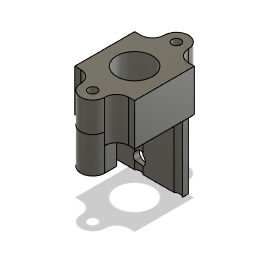
Miniscope_v4_Excitation (Autodesk Fusion 360 design; units mm, degrees)
Autodesk Fusion 360 part; units mm, degrees
sketch "Sketch1" plane through (0, 0, 0) normal (0, 1, 0) x (1, 0, 0)
  line L0 (-1.75, -2.5) -> (1.75, -2.5)
  line L1 (1.75, -2.5) -> (1.75, 2.5)
  line L2 (1.75, 2.5) -> (-1.75, 2.5)
  line L3 (-1.75, 2.5) -> (-1.75, -2.5)
  line L4 (-1.75, -2.5) -> (1.75, 2.5) construction
  line L5 (1.75, -2.5) -> (-1.75, 2.5) construction
  dimension "d1" = 5
  dimension "d2" = 3.5
  constraint perpendicular L0 L1
  constraint parallel L0 L2
  constraint parallel L1 L3
  constraint horizontal L0
  constraint coincident L4 origin
  constraint coincident L5 origin
  measures "d1" distance of L0.end L1.end
  measures "d2" distance of L1.end L2.end
sketch "Sketch2" plane through (0, 0, 0) normal (0, 1, 0) x (1, 0, 0)
  line L0 (-2.5, -2.5) -> (2.5, -2.5)
  line L1 (2.5, -2.5) -> (2.5, 2.5)
  line L2 (2.5, 2.5) -> (-2.5, 2.5)
  line L3 (-2.5, 2.5) -> (-2.5, -2.5)
  line L4 (-2.5, -2.5) -> (2.5, 2.5) construction
  line L5 (2.5, -2.5) -> (-2.5, 2.5) construction
  dimension "d5" = 5
  dimension "d6" = 5
  constraint perpendicular L0 L1
  constraint parallel L0 L2
  constraint parallel L1 L3
  constraint horizontal L0
  constraint coincident L4 origin
  constraint coincident L5 origin
  measures "d5" distance of L1.end L2.end
  measures "d6" distance of L0.end L1.end
extrude "Extrude2" add sketch "Sketch2" along normal blind 3.5
sketch "Sketch3" plane through (0, 3.5, 0) normal (0, 1, 0) x (-1, 0, 0)
  line L0 (2.5, -2.5) -> (2.5, 2.5)
  line L1 (2.5, 2.5) -> (-2.5, 2.5)
  line L2 (-2.5, 2.5) -> (-2.5, -2.5)
  line L3 (-2.5, -2.5) -> (2.5, -2.5)
  circle A0 centre (0, 0) radius 1.5
  dimension "d9" = 3
  constraint coincident A0.centre origin
  measures "d9" diameter of A0
extrude "Extrude3" cut sketch "Sketch3" against normal blind 5 contours A0
sketch "Sketch4" plane through (0, 0, 0) normal (0, -1, 0) x (1, 0, 0)
  circle A0 centre (0, 0) radius 1.5
  line L0 (-2.5, 2.5) -> (-2.5, -2.5)
  line L1 (-2.5, -2.5) -> (2.5, -2.5)
  line L2 (2.5, -2.5) -> (2.5, 2.5)
  line L3 (2.5, 2.5) -> (-2.5, 2.5)
  line L4 (-1.2929, -2) -> (1.2929, -2)
  line L5 (2, -1.2929) -> (2, 1.2929)
  line L6 (1.2929, 2) -> (-1.2929, 2)
  line L7 (-2, 1.2929) -> (-2, -1.2929)
  line L8 (-2, -2) -> (2, 2) construction
  line L9 (2, -2) -> (-2, 2) construction
  arc A1 (-1.2929, 2) -> (-2, 1.2929) centre (-1.6464, 1.6464) ccw
  arc A2 (-2, -1.2929) -> (-1.2929, -2) centre (-1.6464, -1.6464) ccw
  arc A3 (1.2929, -2) -> (2, -1.2929) centre (1.6464, -1.6464) ccw
  arc A4 (2, 1.2929) -> (1.2929, 2) centre (1.6464, 1.6464) ccw
  point P0 (-2, -2)
  point P1 (2, -2)
  point P2 (2, 2)
  dimension "d12" = 4
  dimension "d13" = 4
  dimension "d14" = 1
  constraint perpendicular L4 L5
  constraint parallel L4 L6
  constraint parallel L5 L7
  constraint horizontal L4
  constraint coincident L8 A0.centre
  constraint coincident L9 A0.centre
  constraint coincident A0.centre origin
  constraint coincident L9 A1.centre
  constraint coincident L9.end A1
  measures "d12" distance of P1 P2
  measures "d13" distance of P2 L9.end
  measures "d14" diameter of A1
extrude "Extrude4" cut sketch "Sketch4" against normal blind 1 contours L4 L5 L6 L7 A1 A2 A3 A4
sketch "Sketch5" plane through (0, 0, 0) normal (0, -1, 0) x (1, 0, 0)
  line L0 (-1.2929, 2) -> (1.2929, 2)
  arc A0 (2, 1.2929) -> (1.2929, 2) centre (1.6464, 1.6464) ccw
  line L1 (2, 1.2929) -> (2, -1.2929)
  arc A1 (1.2929, -2) -> (2, -1.2929) centre (1.6464, -1.6464) ccw
  line L2 (1.2929, -2) -> (-1.2929, -2)
  arc A2 (-2, -1.2929) -> (-1.2929, -2) centre (-1.6464, -1.6464) ccw
  line L3 (-2, -1.2929) -> (-2, 1.2929)
  arc A3 (-1.2929, 2) -> (-2, 1.2929) centre (-1.6464, 1.6464) ccw
  line L4 (-2.5, 2.5) -> (-2.5, -2.5)
  line L5 (-2.5, -2.5) -> (2.5, -2.5)
  line L6 (2.5, -2.5) -> (2.5, 2.5)
  line L7 (2.5, 2.5) -> (-2.5, 2.5)
  line L8 (1, 2.5) -> (1, 4.5)
  line L9 (1, 4.5) -> (-1, 4.5)
  line L10 (-1, 4.5) -> (-1, 2.5)
  line L11 (-1, 2.5) -> (1, 4.5) construction
  line L12 (1, 2.5) -> (-1, 4.5) construction
  line L13 (0, 0) -> (0, 3.5) construction
  circle A4 centre (0, 3.5) radius 0.375
  point P0 (0, 3.5)
  dimension "d19" = 2
  dimension "d20" = 2
  dimension "d23" = 0.75
  constraint parallel L8 L10
  constraint coincident L7 L10.end
  constraint coincident L11 P0
  constraint coincident L12 P0
  constraint coincident L13.start origin
  constraint coincident P0 L13.end
  constraint perpendicular L0 L13
  measures "d19" distance of L10.end L9.end
  measures "d20" distance of L8.end L9.end
  measures "d23" diameter of A4
extrude "Extrude5" add sketch "Sketch5" against normal blind 1 contours L7 L8 L9 L10
fillet "Fillet1" radius 1 4 edges at (1, 0.5, 4.5) (1, 0.5, 2.5) (-1, 0.5, 4.5) (-1, 0.5, 2.5)
sketch "Sketch6" plane through (0, 0, 0) normal (0, -1, 0) x (1, 0, 0)
  arc A0 (1, 3.5) -> (-1, 3.5) centre (0, 3.5) ccw
  arc A1 (-2, 2.5) -> (-1, 3.5) centre (-2, 3.5) ccw
  line L0 (-2, 2.5) -> (-2.5, 2.5)
  line L1 (-2.5, 2.5) -> (-2.5, -2.5)
  line L2 (-2.5, -2.5) -> (2.5, -2.5)
  line L3 (2.5, -2.5) -> (2.5, 2.5)
  line L4 (2.5, 2.5) -> (2, 2.5)
  arc A2 (1, 3.5) -> (2, 2.5) centre (2, 3.5) ccw
  circle A3 centre (0, 3.5) radius 0.375
  line L5 (-1.2929, 2) -> (1.2929, 2)
  arc A4 (2, 1.2929) -> (1.2929, 2) centre (1.6464, 1.6464) ccw
  line L6 (2, 1.2929) -> (2, -1.2929)
  arc A5 (1.2929, -2) -> (2, -1.2929) centre (1.6464, -1.6464) ccw
  line L7 (1.2929, -2) -> (-1.2929, -2)
  arc A6 (-2, -1.2929) -> (-1.2929, -2) centre (-1.6464, -1.6464) ccw
  line L8 (-2, -1.2929) -> (-2, 1.2929)
  arc A7 (-1.2929, 2) -> (-2, 1.2929) centre (-1.6464, 1.6464) ccw
  line L9 (-3.6, -2.5) -> (2, -2.5)
  line L10 (2, -2.5) -> (2, -2)
  line L11 (2, -2) -> (-3.6, -2)
  line L12 (-3.6, -2) -> (-3.6, -2.5)
  dimension "d25" = 0.5
  dimension "d30" = 0.5
  dimension "d31" = 1.1
  constraint horizontal L9
  constraint vertical L10
  constraint horizontal L11
  constraint vertical L12
  constraint coincident L2 L9.start
  measures "d25" distance of L9.start L11.end
  measures "d30" distance of L3 L10
  measures "d31" distance of L1 L12
extrude "Extrude6" add sketch "Sketch6" along normal blind 6 contours L1 L2 A5 L7 A6 L9 L10 L11 | L1 L9 L11 L12
sketch "Sketch7" plane through (0, 0, -2.5) normal (0, 0, -1) x (-1, 0, 0)
  line L0 (-2.5, 0) -> (-2, 0)
  line L1 (-2, 0) -> (-2, -6)
  line L2 (-2, -6) -> (3.6, -6)
  line L3 (3.6, -6) -> (3.6, 0)
  line L4 (3.6, 0) -> (2.5, 0)
  line L5 (2.5, 0) -> (2.5, 3.5)
  line L6 (2.5, 3.5) -> (-2.5, 3.5)
  line L7 (-2.5, 3.5) -> (-2.5, 0)
  circle A0 centre (1.6, -5) radius 0.5
  dimension "d35" = 1
  dimension "d37" = 2
  dimension "d38" = 1
  measures "d35" diameter of A0
  measures "d37" distance of L3 A0.centre
  measures "d38" distance of L2 A0.centre
extrude "Extrude7" cut sketch "Sketch7" against normal blind 1 contours A0
sketch "Sketch9" plane through (0, 0, 0) normal (0, -1, 0) x (1, 0, 0)
  line L0 (2, -2) -> (2, -2.5)
  line L1 (2, -2.5) -> (2.5, -2.5)
  line L2 (2.5, -2.5) -> (2.5, 2.5)
  line L3 (2.5, 2.5) -> (2, 2.5)
  arc A0 (1, 3.5) -> (2, 2.5) centre (2, 3.5) ccw
  arc A1 (1, 3.5) -> (-1, 3.5) centre (0, 3.5) ccw
  arc A2 (-2, 2.5) -> (-1, 3.5) centre (-2, 3.5) ccw
  line L4 (-2, 2.5) -> (-2.5, 2.5)
  line L5 (-2.5, 2.5) -> (-2.5, -2)
  line L6 (-2.5, -2) -> (-2, -2)
  arc A3 (-2, -1.2929) -> (-2, -2) centre (-1.6464, -1.6464) ccw
  line L7 (-2, -1.2929) -> (-2, 1.2929)
  arc A4 (-1.2929, 2) -> (-2, 1.2929) centre (-1.6464, 1.6464) ccw
  line L8 (-1.2929, 2) -> (1.2929, 2)
  arc A5 (2, 1.2929) -> (1.2929, 2) centre (1.6464, 1.6464) ccw
  line L9 (2, 1.2929) -> (2, -1.2929)
  arc A6 (2, -2) -> (2, -1.2929) centre (1.6464, -1.6464) ccw
  circle A7 centre (0, 3.5) radius 0.375
  line L10 (-1, 3.5) -> (-1, 2.5)
  line L11 (-1, 2.5) -> (1, 2.5)
  line L12 (1, 2.5) -> (1, 3.5)
  constraint coincident A1.end A2.end
  constraint tangent A1 L10
  constraint perpendicular L10 L11
  constraint coincident A0.start A1.start
  constraint tangent A1 L12
  constraint collinear L3 L11
extrude "Extrude9" add sketch "Sketch9" along normal blind 2 contours A1 L10 L11 L12
sketch "Sketch10" plane through (0, 3.5, 0) normal (0, 1, 0) x (-1, 0, 0)
  circle A0 centre (0, 0) radius 1.5
  line L0 (2.5, -2.5) -> (2.5, 2.5)
  line L1 (2.5, 2.5) -> (-2.5, 2.5)
  line L2 (-2.5, 2.5) -> (-2.5, -2.5)
  line L3 (-2.5, -2.5) -> (2.5, -2.5)
  line L4 (1, -2.5) -> (-1, -2.5)
  line L5 (-1, -2.5) -> (-1, -4.5)
  line L6 (-1, -4.5) -> (1, -4.5)
  line L7 (1, -4.5) -> (1, -2.5)
  line L8 (1, -2.5) -> (-1, -4.5) construction
  line L9 (-1, -2.5) -> (1, -4.5) construction
  line L10 (1, 2.5) -> (-1, 2.5)
  line L11 (-1, 2.5) -> (-1, 4.5)
  line L12 (-1, 4.5) -> (1, 4.5)
  line L13 (1, 4.5) -> (1, 2.5)
  line L14 (1, 2.5) -> (-1, 4.5) construction
  line L15 (-1, 2.5) -> (1, 4.5) construction
  line L16 (0, 0) -> (0, -3.5) construction
  line L17 (0, 0) -> (0, 3.5) construction
  circle A1 centre (0, -3.5) radius 0.375
  circle A2 centre (0, 3.5) radius 0.375
  point P0 (0, -3.5)
  point P1 (0, 3.5)
  dimension "d49" = 2
  dimension "d50" = 2
  dimension "d51" = 2
  dimension "d52" = 2
  dimension "d53" = 0.75
  dimension "d54" = 0.75
  constraint perpendicular L4 L5
  constraint parallel L4 L6
  constraint parallel L5 L7
  constraint horizontal L4
  constraint coincident L3 L4.start
  constraint coincident L8 P0
  constraint coincident L9 P0
  constraint perpendicular L10 L11
  constraint parallel L10 L12
  constraint parallel L11 L13
  constraint horizontal L10
  constraint coincident L1 L10.start
  constraint coincident L14 P1
  constraint coincident L15 P1
  constraint coincident A0.centre L16.start
  constraint coincident P0 L16.end
  constraint vertical L16
  constraint coincident P1 L17.end
  constraint vertical L17
  measures "d49" distance of L4.end L5.end
  measures "d50" distance of L5.end L6.end
  measures "d51" distance of L10.start L12.end
  measures "d52" distance of L11.end L12.end
  measures "d53" diameter of A1
  measures "d54" diameter of A2
extrude "Extrude10" add sketch "Sketch10" against normal blind 2.5 contours L3 L4 L5 L6 L7 | L1 L10 L11 L12 L13
fillet "Fillet2" radius 1 8 edges at (1, 2.25, 4.5) (-1, 2.25, 4.5) (-1, 2.25, 2.5) (-1, 2.25, -4.5) (-1, 2.25, -2.5) (1, 2.25, -4.5) (1, 2.25, -2.5) (1, 2.25, 2.5)
